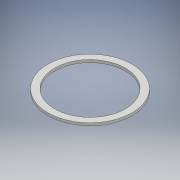
# Autodesk Inventor part: Medio Circulo
Saved by Autodesk Inventor 2018 (Build 220112000, 112)
## iProperties
Created: 2018-04-04
Part Number: Medio Circulo
Material: Générique
Document SubType Name: Modeling
Designer: Guadalix
Density: 1 g/cm^3
Appearance: Par défaut
Author: Guadalix
Autodesk Inventor part; units mm, degrees
ref_plane "YZ Plane" through (0, 0, 0) normal (1, 0, 0) x (0, 1, 0)
ref_plane "XZ Plane" through (0, 0, 0) normal (0, 1, 0) x (-1, 0, 0)
ref_plane "XY Plane" through (0, 0, 0) normal (0, 0, 1) x (1, 0, 0)
sketch "Esquisse1" plane through (0, 0, 0) normal (0, 0, 1) x (1, 0, 0)
  circle A0 centre (0, 0) radius 47.5
  circle A1 centre (0, 0) radius 40
  point P0 (0, 45)
  point P1 (0, 47.5)
  dimension "d0" = 95
  dimension "d1" = 80
  dimension "d2" = 2.5
  constraints: 2 coincident, 1 centre point, 1 vertical alignment, 2 other
  measures "d1" diameter of A1
  measures "d2" distance of point (0, 45) point (0, 47.5)
sketch "Esquisse2" plane through (0, 0, 0) normal (0, 0, 1) x (1, 0, 0)
  circle A0 centre (0, 43.6003) radius 3.0751
  point P0 (0, 0)
  constraints: 1 centre point
extrude "Extrusion1" add sketch "Esquisse1" along normal blind 3
extrude "Extrusion2" cut sketch "Esquisse2" along normal blind 2
